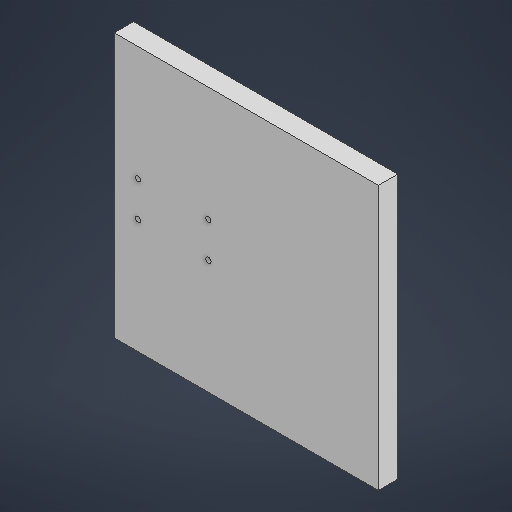
# Autodesk Inventor part: Teste bloco do motor
Saved by Autodesk Inventor 2026.1 (Build 301233020, 233B)
## iProperties
Created: 2026-03-18
Part Number: Teste bloco do motor
Material: Generic
Document SubType Name: Modeling
Designer: 062210040
Density: 1 g/cm^3
Appearance: Default
Author: 062210040
Autodesk Inventor part; units mm, degrees
ref_plane "YZ Plane" through (0, 0, 0) normal (1, 0, 0) x (0, 1, 0)
ref_plane "XZ Plane" through (0, 0, 0) normal (0, 1, 0) x (-1, 0, 0)
ref_plane "XY Plane" through (0, 0, 0) normal (0, 0, 1) x (1, 0, 0)
sketch "Sketch1" plane through (0, 0, 0) normal (0, 0, 1) x (1, 0, 0)
  line L0 (0, 0) -> (150, 0)
  line L1 (150, 0) -> (150, 150)
  line L2 (150, 150) -> (0, 150)
  line L3 (0, 150) -> (0, 0)
  dimension "d0" = 150
  dimension "d1" = 150
  constraints: 8 end point, 2 parallel, 1 horizontal, 1 perpendicular
  measures "d0" distance of L2.end L1.end
  measures "d1" distance of L1.end L0.end
extrude "Extrusion1" add sketch "Sketch1" along normal blind 11
sketch "Sketch2" plane through (0, 0, 11) normal (0, 0, 1) x (1, 0, 0)
  circle A0 centre (13.5, 85) radius 1.5
  circle A1 centre (13.5, 65) radius 1.5
  circle A2 centre (53.5, 85) radius 1.5
  circle A3 centre (53.5, 65) radius 1.5
  line L0 (0, 150) -> (0, 0) projected
  line L1 (0, 0) -> (150, 0) projected
  line L2 (150, 150) -> (0, 150) projected
  line L3 (75, 150) -> (75, 0)
  line L4 (-23.1394, 75) -> (177.6706, 75)
  dimension "d4" = 3
  dimension "d5" = 3
  dimension "d6" = 20
  dimension "d7" = 3
  dimension "d8" = 3
  dimension "d10" = 40
  dimension "d11" = 40
  dimension "d12" = 20
  dimension "d13" = 13.5
  dimension "d14" = 13.5
  dimension "d15" = 65
  dimension "d16" = 65
  constraints: 4 centre point, 4 end point, 2 horizontal, 2 midpoint
  measures "d4" diameter of A0
  measures "d5" diameter of A1
  measures "d6" distance of A0.centre A1.centre
  measures "d7" diameter of A2
  measures "d8" diameter of A3
  measures "d10" distance of A1.centre A3.centre
  measures "d11" distance of A2.centre A0.centre
  measures "d12" distance of A3.centre A2.centre
  measures "d13" distance from line of L0 A0.centre
  measures "d14" distance from line of L0 A1.centre
  measures "d15" distance from line of L1 A1.centre
  measures "d16" distance from line of L1 A3.centre
extrude "Extrusion2" cut sketch "Sketch2" against normal blind 11 contours A0 | A1 | A2 | A3
body "Solid1"
